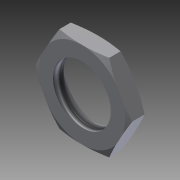
# Autodesk Inventor part: AT513H
Saved by Autodesk Inventor 2014 (Build 180170000, 170)
## iProperties
Category: PARTsolutions
Company: NKKSWITCHES
Created: 2013-12-29
Part Number: AT513H
Catalog Web Link: www.cadenas.de
Description: Hex Nut - Bushing Mount Miniature Toggles-Series M - Standard Hardwarw for Small & Large Bushings
Vendor: NKKSWITCHES
Document SubType Name: Modeling
Designer: PARTuser1
Manufacturer: NKKSWITCHES
Density: 1 g/cm^3
Material: Generic
Appearance: RGB(192.00000375509219,192.00000375509219,192.00000375509219)
PSOL_IDENT_0: {$CADENAS_DATA\23d-libs\nkkswitches\toggle\m\hardware\hex_nut.prj},189 {VTYP=3D},{NB=AT513H},{LINA=A
PSOL_IDENT_1: T513H},{NN=Hex Nut - Bushing Mount Miniature Toggles},{DATE=07.12.2009 12:30:45},{GEOMDATE=07.12.200
PSOL_IDENT_2: 9 11:39:00},{VERSION=},{LINEID=10},{LINESUBID=-1},{WBVAR=}  {NB=AT513H},{LINA=AT513H},{KT=DUMMY},{PN
PSOL_IDENT_3: =AT513H},{S=0.315},{D=1/4-40},{DMAX=0.25},{DMIN=0.22},{T=0.059},{W=0.354}
CNS_NN: Hex Nut - Bushing Mount Miniature Toggles
CNS_NT: Series M - Standard Hardwarw for Small & Large Bushings
CNS_NB: AT513H
CNS_NBSYN: $PN.
CNS_LINA: AT513H
CNS_PN: AT513H
CNS_S: 0.315
CNS_D: 1/4-40
CNS_DMAX: 0.25
CNS_DMIN: 0.22
CNS_T: 0.059
CNS_W: 0.354
SUPPLIER: NKKSWITCHES
ARTICLENO: AT513H
BOMINFO: AT513H
CREATOR: CADENAS GmbH
Title: AT513H
Author: Cadenas PARTsolutions
Comments: Series M - Standard Hardwarw for Small & Large Bushings
Autodesk Inventor part; units mm, degrees
sketch "Sketch_1" plane through (0, 0, 0) normal (1, 0, 0) x (0, 1, 0)
  line L0 (0, -0.7493) -> (0, 0.7493)
  line L1 (0, 0.7493) -> (4.0005, 0.7493)
  line L2 (4.0005, 0.7493) -> (4.8006, 0.4581)
  line L3 (4.8006, 0.4581) -> (4.8006, -0.4581)
  line L4 (4.8006, -0.4581) -> (4.0005, -0.7493)
  line L5 (4.0005, -0.7493) -> (0, -0.7493)
  line L6 (0, -0.7493) -> (0, 0.7493)
  constraints: 14 end point
revolve "Revolution1" add sketch "Sketch_1" angle 360 about axis through (0, 0, -0.7493) along (0, 0, -1)
sketch "Sketch_2" plane through (0, 0, 0) normal (0, 0, 1) x (1, 0, 0)
  line L0 (-8.001, 8.001) -> (-8.001, -8.001)
  line L1 (-8.001, -8.001) -> (8.001, -8.001)
  line L2 (8.001, -8.001) -> (8.001, 8.001)
  line L3 (8.001, 8.001) -> (-8.001, 8.001)
  line L4 (-4.4958, 0) -> (-2.3097, -4.0005)
  line L5 (-2.3097, -4.0005) -> (2.3097, -4.0005)
  line L6 (2.3097, -4.0005) -> (4.4958, 0)
  line L7 (4.4958, 0) -> (2.3097, 4.0005)
  line L8 (2.3097, 4.0005) -> (-2.3097, 4.0005)
  line L9 (-2.3097, 4.0005) -> (-4.4958, 0)
  constraints: 20 end point
extrude "Extrusion1" cut sketch "Sketch_2" along normal mid plane 2.9972
sketch "Sketch3" plane through (0, 0, -0.7493) normal (0, 0, -1) x (-1, 0, 0)
  point P0 (0, 0)
hole "Drilling 1" at (0, 0, -0.7493) direction (0, 0, 1) diameter 5.3594 depth 1.4986 countersink diameter 6.35 countersink angle 90 thread size "1/4-28 UNF" class "2B" standard "ANSI Unified Screw Threads"
ref_plane "nut_XY" through (0, 0, 0.7493) normal (0, 0, 1) x (1, 0, 0)
ref_plane "nut_YZ" through (0, 0, 0.7493) normal (1, 0, 0) x (0, 1, 0)
ref_plane "nut_ZX" through (0, 0, 0.7493) normal (0, 1, 0) x (0, 0, 1)
body "Solid1"
